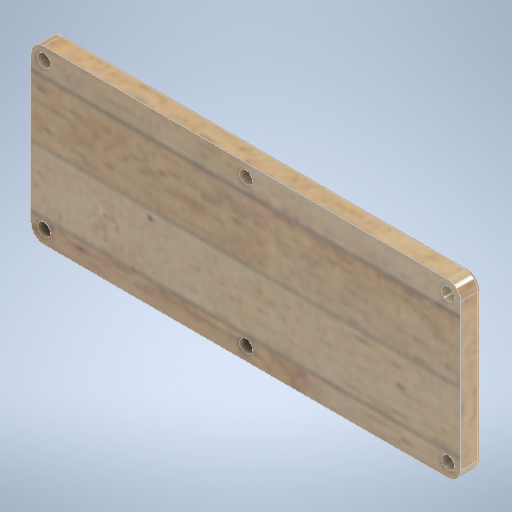
# Autodesk Inventor part: 35 - Wooden Base
Saved by Autodesk Inventor 2025.2 (Build 292293000, 293)
## iProperties
Created: 2025-07-30
Part Number: 35 - Wooden Base
Material: Wood (Maple)
Document SubType Name: Modeling
Designer: bless
Density: 0.67 g/cm^3
Appearance: Natural Maple - Glossy Dark Tint
Author: bless
Autodesk Inventor part; units mm, degrees
ref_plane "YZ Plane" through (0, 0, 0) normal (1, 0, 0) x (0, 1, 0)
ref_plane "XZ Plane" through (0, 0, 0) normal (0, 1, 0) x (-1, 0, 0)
ref_plane "XY Plane" through (0, 0, 0) normal (0, 0, 1) x (1, 0, 0)
sketch "Sketch1" plane through (0, 0, 0) normal (0, 0, 1) x (1, 0, 0)
  line L0 (0, 0) -> (400, 0)
  line L1 (400, 0) -> (400, 160)
  line L2 (400, 160) -> (0, 160)
  line L3 (0, 160) -> (0, 0)
  dimension "d0" = 400
  dimension "d1" = 160
  constraints: 8 end point, 2 parallel, 1 horizontal, 1 perpendicular
  measures "d0" distance of L0.start L0.end
  measures "d1" distance of L2.end L0.start
extrude "Extrusion1" add sketch "Sketch1" against normal blind 19
fillet "Fillet1" radius 12 4 edges at (400, 160, -9.5) (400, 0, -9.5) (0, 0, -9.5) (0, 160, -9.5)
fillet "Fillet2" radius 3 8 edges at (3.5147, 3.5147, -19) (0, 80, -19) (3.5147, 156.4853, -19) (200, 160, -19) (396.4853, 156.4853, -19) (400, 80, -19) (396.4853, 3.5147, -19) (200, 0, -19)
sketch "Sketch3" plane through (0, 0, 0) normal (0, 0, 1) x (1, 0, 0)
  arc A0 (12, 160) -> (0, 148) centre (12, 148) ccw projected
  line L0 (0, 148) -> (0, 12) projected
  arc A1 (0, 12) -> (12, 0) centre (12, 12) ccw projected
  arc A2 (388, 0) -> (400, 12) centre (388, 12) ccw projected
  line L1 (400, 12) -> (400, 148) projected
  arc A3 (400, 148) -> (388, 160) centre (388, 148) ccw projected
  point P0 (0, 0)
  point P1 (200, 148)
  point P2 (200, 12)
  point P3 (0, 80)
  point P4 (400, 80)
  dimension "d18" = 188
  dimension "d19" = 188
  dimension "d20" = 68
  dimension "d21" = 68
  constraints: 4 coincident, 2 midpoint
  measures "d18" distance of point (200, 148) point (12, 148)
  measures "d19" distance of point (388, 12) point (200, 12)
  measures "d20" vertical distance of point (0, 80) point (200, 148)
  measures "d21" vertical distance of point (400, 80) point (200, 12)
hole "Hole2" at (12, 148, 0) at (200, 148, 0) at (388, 148, 0) at (388, 12, 0) at (200, 12, 0) at (12, 12, 0) direction (0, 0, -1) diameter 5.5 end through all counterbore diameter 12 counterbore depth 8
body "Solid1"
